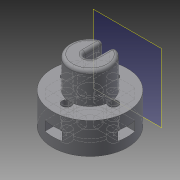
# Autodesk Inventor part: screwServo
Saved by Autodesk Inventor 2015 (Build 190159000, 159)
## iProperties
Created: 2016-10-16
Part Number: screwServo
Material: Generic
Document SubType Name: Modeling
Designer: Bardo91
Density: 1 g/cm^3
Appearance: Default
Author: Bardo91
Autodesk Inventor part; units mm, degrees
ref_plane "YZ Plane" through (0, 0, 0) normal (1, 0, 0) x (0, 1, 0)
ref_plane "XY Plane" through (0, 0, 0) normal (0, 0, 1) x (1, 0, 0)
sketch "Sketch1" plane through (0, 0, 0) normal (0, 0, 1) x (1, 0, 0)
  line L0 (0, 0) -> (0, 7.5)
  circle A0 centre (0, 7.5) radius 1.5
  circle A1 centre (-5.3033, 5.3033) radius 1.5
  circle A2 centre (-7.5, 0) radius 1.5
  circle A3 centre (-5.3033, -5.3033) radius 1.5
  circle A4 centre (0, -7.5) radius 1.5
  circle A5 centre (5.3033, -5.3033) radius 1.5
  circle A6 centre (7.5, 0) radius 1.5
  circle A7 centre (5.3033, 5.3033) radius 1.5
  circle A8 centre (0, 0) radius 12
  dimension "d0" = 7.5
  dimension "d1" = 3
  dimension "d4" = 360
  dimension "d6" = 24
  constraints: 9 centre point, 2 coincident, 2 end point, 1 vertical, 17 other
  measures "d0" distance of L0.start L0.end
  measures "d1" diameter of A0
  measures "d6" diameter of A8
extrude "Extrusion1" add sketch "Sketch1" along normal blind 10 contours A1 | A3 | A5 | A7 | A8
sketch "Sketch2" plane through (0, 0, 0) normal (0, 0, -1) x (-1, 0, 0)
  circle A0 centre (0, 0) radius 6.5
  dimension "d9" = 13
  constraints: 1 centre point, 1 coincident
  measures "d9" diameter of A0
extrude "Extrusion2" cut sketch "Sketch2" against normal blind 1
sketch "Sketch3" plane through (0, 0, 10) normal (0, 0, 1) x (1, 0, 0)
  circle A0 centre (0, 0) radius 6.5
  dimension "d12" = 13
  constraints: 1 centre point, 1 coincident
  measures "d12" diameter of A0
extrude "Extrusion3" add sketch "Sketch3" along normal blind 10
sketch "Sketch4" plane through (0, 0, 10) normal (0, 0, 1) x (1, 0, 0)
  line L0 (0, 0) -> (-6.5, 0)
  circle A0 centre (0, 0) radius 6.5 projected
  line L1 (0, 0) -> (-3.5, 0)
  line L2 (-3.5, 0) -> (3.5, 0)
  line L3 (3.5, 0) -> (3.5, -3)
  line L4 (1.75, 3.0311) -> (4.3481, 1.5311)
  line L5 (-1.75, 3.0311) -> (0.8481, 4.5311)
  line L6 (-3.5, 0) -> (-3.5, 3)
  line L7 (-1.75, -3.0311) -> (-4.3481, -1.5311)
  line L8 (1.75, -3.0311) -> (-0.8481, -4.5311)
  line L9 (0, 0) -> (0, -4.0415)
  line L10 (0, 0) -> (0, 4.0415)
  line L11 (3.5, 0) -> (3.5, 2.0207)
  line L12 (0, 4.0415) -> (1.75, 3.0311)
  line L13 (-1.75, 3.0311) -> (-3.5, 2.0207)
  line L14 (-3.5, 0) -> (-3.5, -2.0207)
  line L15 (-1.75, -3.0311) -> (0, -4.0415)
  line L16 (1.75, -3.0311) -> (3.5, -2.0207)
  line L17 (3.5, 2.0207) -> (3.5, 7.0207)
  line L18 (3.5, 7.0207) -> (-3.5, 7.0207)
  line L19 (-3.5, 7.0207) -> (-3.5, 3)
  dimension "d15" = 3.5
  dimension "d16" = 7
  dimension "d17" = 3
  dimension "d20" = 360
  dimension "d22" = 5
  constraints: 40 end point, 9 point on line, 4 parallel, 3 vertical, 2 perpendicular, 1 horizontal alignment, 20 other
  measures "d15" distance of L0.start L1.end
  measures "d16" distance of L1.end L2.end
  measures "d17" distance of L2.end L3.end
  measures "d22" distance of L11.end L17.end
extrude "Extrusion4" cut sketch "Sketch4" along normal blind 6 contours L9 L15 L7 L14 L0 | L10 L12 L4 L11 L2 | L2 L3 L16 L8 L9 | L0 L6 L13 L5 L10 | L5 L13 L6 L19 A0 L17 L4 L12 | L19 L18 L17 A0
sketch "Sketch5" plane through (0, 0, 20) normal (0, 0, 1) x (1, 0, 0)
  circle A0 centre (0, 0) radius 1.5
  dimension "d25" = 3
  constraints: 1 centre point, 1 coincident
  measures "d25" diameter of A0
extrude "Extrusion5" cut sketch "Sketch5" against normal up to surface (19 mm away)
sketch "Sketch6" plane through (0, 0, 20) normal (0, 0, 1) x (1, 0, 0)
  circle A0 centre (0, 0) radius 1.5 projected
  line L0 (1.5, 0) -> (1.5, 15)
  line L1 (1.5, 0) -> (-1.5, 0)
  line L2 (-1.5, 0) -> (-1.5, 15)
  line L3 (-1.5, 15) -> (1.5, 15)
  dimension "d28" = 15
  dimension "d29" = 15
  constraints: 8 end point, 2 point on circle, 1 horizontal, 1 perpendicular, 1 tangent, 1 vertical
  measures "d28" distance of L0.start L0.end
  measures "d29" distance of L1.end L2.end
extrude "Extrusion6" cut sketch "Sketch6" against normal up to surface (4 mm away) contours A0 L2 L3 L0
fillet "Fillet1" radius 1 2 edges at (1.5, 6.3246, 18) (-1.5, 6.3246, 18)
fillet "Fillet2" radius 1 6 edges at (1.9778, 5.7518, 20) (1.5, 2.4495, 20) (0, -1.5, 20) (-1.5, 2.4495, 20) (-1.9778, 5.7518, 20) (0, -6.5, 20)
ref_plane "Work Plane1" through (0, 12, 0) normal (0, 1, 0) x (-1, 0, 0)
sketch "Sketch7" plane through (0, 12, 0) normal (0, 1, 0) x (-1, 0, 0)
  line L0 (0, 0) -> (0, 3)
  line L1 (0, 3) -> (2.75, 3)
  line L2 (2.75, 3) -> (2.75, 6)
  line L3 (2.75, 6) -> (-2.75, 6)
  line L4 (-2.75, 6) -> (-2.75, 3)
  line L5 (-2.75, 3) -> (0, 3)
  dimension "d35" = 3
  dimension "d36" = 2.75
  dimension "d37" = 3
  dimension "d38" = 5.5
  constraints: 12 end point, 4 perpendicular, 1 horizontal, 1 vertical
  measures "d35" distance of L0.start L0.end
  measures "d36" distance of L0.end L1.end
  measures "d37" distance of L1.end L2.end
  measures "d38" distance of L2.end L3.end
extrude "Extrusion7" cut sketch "Sketch7" against normal blind 8
pattern_circular "Circular Pattern1" count 4 over 360 about axis through (0, 0, 20) along (0, 0, -1) of "Extrusion7"
sketch "Sketch8" plane through (0, 0, 10) normal (0, 0, 1) x (1, 0, 0)
  circle A0 centre (0, 0) radius 3
  dimension "d44" = 6
  constraints: 1 centre point, 1 coincident
  measures "d44" diameter of A0
extrude "Extrusion8" cut sketch "Sketch8" against normal through all
body "Solid1"
